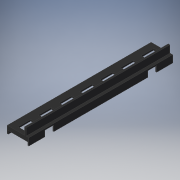
# Autodesk Inventor part: PRO10282 Rollenleiste Abdeckung mit Seitenfuehrung 250
Saved by Autodesk Inventor 2019 (Build 230136000, 136)
## iProperties
Created: 2023-08-22
Part Number: PRO10282 Rollenleiste Abdeckung mit Seitenfuehrung 250
Material: Generic
Catalog Web Link: www.cadenas.de
Description: PRO10282-Roller track cover with side guide
Vendor: ROBOTUNITS
Document SubType Name: Modeling
Designer: psAdmin
Manufacturer: ROBOTUNITS
Mass: 35.939 g
Surface Area: 329.421 cm^2
Volume: 35.939 cm^3
Density: 1 g/cm^3
Appearance: PSOLRGB-175-175-175
Category: PARTsolutions
Company: ROBOTUNITS
Title: PRO10282 Rollenleiste Abdeckung mit Seitenfuehrung 250
Author: Cadenas PARTsolutions
Comments: Roller track cover with side guide
PSOL_IDENT_0: {$CADENAS_DATA/23d-libs/robotunits/mbs_pickstar/parts_materialbereitstellungssystem/pro_10282.prj},2
PSOL_IDENT_1: 52 {VTYP=3D},{NB=PRO10282 Rollenleiste Abdeckung mit Seitenfuehrung 250},{LINA=PRO10282 Rollenleiste
PSOL_IDENT_2: Abdeckung mit Seitenfuehrung 250},{NN=PRO10282},{DATE=25.04.2023 06:52:35},{GEOMDATE=15.02.2017 11:
PSOL_IDENT_3: 51:48},{VERSION=},{LINEID=10},{WBVAR=L},{WBNUMERIC=L}  {NB=PRO10282 Rollenleiste Abdeckung mit Seite
PSOL_IDENT_4: nfuehrung 250},{LINA=PRO10282 Rollenleiste Abdeckung mit Seitenfuehrung 250},{KT=DUMMY},{L=250},{LX=
PSOL_IDENT_5: 0250},{LXX=250,[45:250]},{B=37.500}
NB: PRO10282 Rollenleiste Abdeckung mit Seitenfuehrung 250
NN: PRO10282
NT: Roller track cover with side guide
NBSYN: PRO10282 Rollenleiste Abdeckung mit Seitenfuehrung $L.
LINA: PRO10282 Rollenleiste Abdeckung mit Seitenfuehrung 250
CATALOG: Robotunits
L: 250
B: 37.5
SUPPLIER: ROBOTUNITS
ARTICLENO: PRO10282 Rollenleiste Abdeckung mit Seitenfuehrung 250
BOMINFO: PRO10282 Rollenleiste Abdeckung mit Seitenfuehrung 250
CREATOR: CADENAS GmbH
Autodesk Inventor part; units mm, degrees
ref_plane "YZ Plane" through (0, 0, 0) normal (1, 0, 0) x (0, 1, 0)
ref_plane "XZ Plane" through (0, 0, 0) normal (0, 1, 0) x (-1, 0, 0)
ref_plane "XY Plane" through (0, 0, 0) normal (0, 0, 1) x (1, 0, 0)
sketch "Sketch_1" plane through (0, 0, 0) normal (0, 0, 1) x (1, 0, 0)
  line L0 (-18.75, -12.5) -> (-17, -12.5)
  line L1 (-17, -12.5) -> (-17, -7.2)
  line L2 (-17, -7.2) -> (17, -7.2)
  line L3 (17, -7.2) -> (17, -12.5)
  line L4 (17, -12.5) -> (18.75, -12.5)
  line L5 (18.75, -12.5) -> (18.75, 0)
  line L6 (18.75, 0) -> (14, 0)
  line L7 (14, 0) -> (14, 12.5)
  line L8 (14, 12.5) -> (11, 12.5)
  line L9 (11, 12.5) -> (11, 0)
  line L10 (11, 0) -> (-18.75, 0)
  line L11 (-18.75, 0) -> (-18.75, -12.5)
  constraints: 24 end point
extrude "Extrusion1" add sketch "Sketch_1" along normal blind 250
sketch "Sketch_2" plane through (-18.75, 0, 0) normal (0, 1, 0) x (0, 0, 1)
  line L0 (6.645, 11.65) -> (28.795, 11.65)
  line L1 (28.795, 11.65) -> (28.795, 25.85)
  line L2 (28.795, 25.85) -> (6.645, 25.85)
  line L3 (6.645, 25.85) -> (6.645, 11.65)
  constraints: 8 end point
extrude "Extrusion2" cut sketch "Sketch_2" against normal blind 8
sketch "Sketch_3" plane through (-18.75, 0, 0) normal (0, 1, 0) x (0, 0, 1)
  line L0 (42.355, 25.85) -> (42.355, 11.65)
  line L1 (42.355, 11.65) -> (64.505, 11.65)
  line L2 (64.505, 11.65) -> (64.505, 25.85)
  line L3 (64.505, 25.85) -> (42.355, 25.85)
  constraints: 8 end point
extrude "Extrusion3" cut sketch "Sketch_3" against normal blind 8
sketch "Sketch_4" plane through (-18.75, 0, 0) normal (0, 1, 0) x (0, 0, 1)
  line L0 (78.065, 11.65) -> (100.215, 11.65)
  line L1 (100.215, 11.65) -> (100.215, 25.85)
  line L2 (100.215, 25.85) -> (78.065, 25.85)
  line L3 (78.065, 25.85) -> (78.065, 11.65)
  constraints: 8 end point
extrude "Extrusion4" cut sketch "Sketch_4" against normal blind 8
sketch "Sketch_5" plane through (-18.75, 0, 0) normal (0, 1, 0) x (0, 0, 1)
  line L0 (113.775, 25.85) -> (113.775, 11.65)
  line L1 (113.775, 11.65) -> (135.925, 11.65)
  line L2 (135.925, 11.65) -> (135.925, 25.85)
  line L3 (135.925, 25.85) -> (113.775, 25.85)
  constraints: 8 end point
extrude "Extrusion5" cut sketch "Sketch_5" against normal blind 8
sketch "Sketch_6" plane through (-18.75, 0, 0) normal (0, 1, 0) x (0, 0, 1)
  line L0 (149.485, 25.85) -> (149.485, 11.65)
  line L1 (149.485, 11.65) -> (171.635, 11.65)
  line L2 (171.635, 11.65) -> (171.635, 25.85)
  line L3 (171.635, 25.85) -> (149.485, 25.85)
  constraints: 8 end point
extrude "Extrusion6" cut sketch "Sketch_6" against normal blind 8
sketch "Sketch_7" plane through (-18.75, 0, 0) normal (0, 1, 0) x (0, 0, 1)
  line L0 (185.195, 11.65) -> (207.345, 11.65)
  line L1 (207.345, 11.65) -> (207.345, 25.85)
  line L2 (207.345, 25.85) -> (185.195, 25.85)
  line L3 (185.195, 25.85) -> (185.195, 11.65)
  constraints: 8 end point
extrude "Extrusion7" cut sketch "Sketch_7" against normal blind 8
sketch "Sketch_8" plane through (-18.75, 0, 0) normal (0, 1, 0) x (0, 0, 1)
  line L0 (220.905, 25.85) -> (220.905, 11.65)
  line L1 (220.905, 11.65) -> (243.055, 11.65)
  line L2 (243.055, 11.65) -> (243.055, 25.85)
  line L3 (243.055, 25.85) -> (220.905, 25.85)
  constraints: 8 end point
extrude "Extrusion8" cut sketch "Sketch_8" against normal blind 8
sketch "Sketch_10" plane through (-18.75, -12.5, 0) normal (-1, 0, 0) x (0, 0, 1)
  line L0 (27.9, 10) -> (27.9, 0)
  line L1 (27.9, 0) -> (43.3, 0)
  line L2 (43.3, 0) -> (43.3, 10)
  line L3 (43.3, 10) -> (27.9, 10)
  constraints: 8 end point
extrude "Extrusion9" cut sketch "Sketch_10" against normal blind 37.5
sketch "Sketch_11" plane through (-18.75, -12.5, 0) normal (-1, 0, 0) x (0, 0, 1)
  line L0 (206.7, 10) -> (206.7, 0)
  line L1 (206.7, 0) -> (222.1, 0)
  line L2 (222.1, 0) -> (222.1, 10)
  line L3 (222.1, 10) -> (206.7, 10)
  constraints: 8 end point
extrude "Extrusion10" cut sketch "Sketch_11" against normal blind 37.5
sketch "Sketch_13" plane through (-17, -7.2, 0) normal (0, -1, 0) x (1, 0, 0)
  line L0 (0, 247) -> (0, 3)
  line L1 (0, 3) -> (34, 3)
  line L2 (34, 3) -> (34, 247)
  line L3 (34, 247) -> (0, 247)
  constraints: 8 end point
extrude "Extrusion11" cut sketch "Sketch_13" against normal blind 4.7
ref_plane "p_XY" through (0, 0, 0) normal (0, 1, 0) x (1, 0, 0)
ref_plane "p_YZ" through (0, 0, 0) normal (1, 0, 0) x (0, 0, -1)
ref_plane "p_ZX" through (0, 0, 0) normal (0, 0, -1) x (0, 1, 0)
ref_plane "p1_XY" through (0, -9.5, 17.72) normal (1, 0, 0) x (0, 0, -1)
ref_plane "p1_YZ" through (0, -9.5, 17.72) normal (0, 0, -1) x (0, 1, 0)
ref_plane "p1_ZX" through (0, -9.5, 17.72) normal (0, 1, 0) x (1, 0, 0)
ref_plane "p2_XY" through (0, -9.5, 53.43) normal (1, 0, 0) x (0, 0, -1)
ref_plane "p2_YZ" through (0, -9.5, 53.43) normal (0, 0, -1) x (0, 1, 0)
ref_plane "p2_ZX" through (0, -9.5, 53.43) normal (0, 1, 0) x (1, 0, 0)
ref_plane "p3_XY" through (0, -9.5, 89.14) normal (1, 0, 0) x (0, 0, -1)
ref_plane "p3_YZ" through (0, -9.5, 89.14) normal (0, 0, -1) x (0, 1, 0)
ref_plane "p3_ZX" through (0, -9.5, 89.14) normal (0, 1, 0) x (1, 0, 0)
ref_plane "p4_XY" through (0, -9.5, 124.85) normal (1, 0, 0) x (0, 0, -1)
ref_plane "p4_YZ" through (0, -9.5, 124.85) normal (0, 0, -1) x (0, 1, 0)
ref_plane "p4_ZX" through (0, -9.5, 124.85) normal (0, 1, 0) x (1, 0, 0)
ref_plane "p5_XY" through (0, -9.5, 160.56) normal (1, 0, 0) x (0, 0, -1)
ref_plane "p5_YZ" through (0, -9.5, 160.56) normal (0, 0, -1) x (0, 1, 0)
ref_plane "p5_ZX" through (0, -9.5, 160.56) normal (0, 1, 0) x (1, 0, 0)
ref_plane "p6_XY" through (0, -9.5, 196.27) normal (1, 0, 0) x (0, 0, -1)
ref_plane "p6_YZ" through (0, -9.5, 196.27) normal (0, 0, -1) x (0, 1, 0)
ref_plane "p6_ZX" through (0, -9.5, 196.27) normal (0, 1, 0) x (1, 0, 0)
ref_plane "p7_XY" through (0, -9.5, 231.98) normal (1, 0, 0) x (0, 0, -1)
ref_plane "p7_YZ" through (0, -9.5, 231.98) normal (0, 0, -1) x (0, 1, 0)
ref_plane "p7_ZX" through (0, -9.5, 231.98) normal (0, 1, 0) x (1, 0, 0)
body "Solid1"
